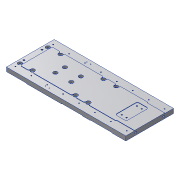
# Autodesk Inventor part: Grundplatte
Saved by Autodesk Inventor 2016 (Build 200138000, 138)
## iProperties
Created: 2015-07-27
Part Number: Grundplatte
Material: Aluminum 6061
Document SubType Name: Modeling
Density: 2.7 g/cm^3
Appearance: Aluminum - Flat
Autodesk Inventor part; units mm, degrees
ref_plane "YZ Plane" through (0, 0, 0) normal (1, 0, 0) x (0, 1, 0)
ref_plane "XZ Plane" through (0, 0, 0) normal (0, 1, 0) x (-1, 0, 0)
ref_plane "XY Plane" through (0, 0, 0) normal (0, 0, 1) x (1, 0, 0)
sketch "Sketch1" plane through (0, 0, 0) normal (0, 0, 1) x (1, 0, 0)
  line L0 (-150, -60) -> (150, -60)
  line L1 (150, -60) -> (150, 60)
  line L2 (150, 60) -> (-150, 60)
  line L3 (-150, 60) -> (-150, -60)
  line L4 (-150, -60) -> (150, 60) construction
  line L5 (150, -60) -> (-150, 60) construction
  point P0 (0, 0)
  dimension "d0" = 300
  dimension "d1" = 120
  constraints: 12 end point, 2 midpoint, 2 parallel, 1 horizontal, 1 perpendicular
  measures "d0" distance of L2.end L1.end
  measures "d1" distance of L1.end L0.end
extrude "Extrusion1" add sketch "Sketch1" along normal blind 12
sketch "Sketch2" plane through (0, 0, 12) normal (0, 0, 1) x (1, 0, 0)
  line L0 (150, -60) -> (-150, -60)
  line L1 (-150, -60) -> (-150, -40)
  line L2 (-150, -40) -> (150, -40)
  line L3 (150, -40) -> (150, -60)
  line L4 (150, 60) -> (-150, 60)
  line L5 (-150, 60) -> (-150, 40)
  line L6 (-150, 40) -> (150, 40)
  line L7 (150, 40) -> (150, 60)
  line L8 (-135, 40) -> (-150, 40)
  line L9 (-150, 40) -> (-150, -40)
  line L10 (-150, -40) -> (-135, -40)
  line L11 (-135, -40) -> (-135, 40)
  line L12 (150, -60) -> (150, 60) projected
  line L13 (-150, -60) -> (150, -60) projected
  line L14 (-150, 60) -> (-150, -60) projected
  line L15 (150, 60) -> (-150, 60) projected
  line L16 (119, 28) -> (91, 28)
  line L17 (91, 28) -> (91, -28)
  line L18 (91, -28) -> (119, -28)
  line L19 (119, -28) -> (119, 28)
  line L20 (150, -40) -> (105, -40)
  line L21 (105, -40) -> (105, -38)
  line L22 (105, -38) -> (150, -38)
  line L23 (150, -38) -> (150, -40)
  line L24 (150, 40) -> (105, 40)
  line L25 (105, 40) -> (105, 38)
  line L26 (105, 38) -> (150, 38)
  line L27 (150, 38) -> (150, 40)
  point P0 (0, 0)
  point P1 (91, 0)
  dimension "d4" = 80
  dimension "d5" = 15
  dimension "d6" = 269
  dimension "d7" = 28
  dimension "d8" = 56
  dimension "d26" = 2
  dimension "d134" = 255
  constraints: 48 end point, 12 parallel, 9 collinear, 6 horizontal, 6 perpendicular, 1 horizontal alignment, 1 midpoint, 1 point on line
  measures "d4" distance between parallel lines of L6 L2
  measures "d5" distance between parallel lines of L9 L11
  measures "d6" distance between parallel lines of L14 L19
  measures "d7" distance of L17.end L18.end
  measures "d8" distance of L18.end L16.start
  measures "d26" distance of L20.end L21.end
  measures "d134" distance between parallel lines of L1 L21
extrude "Extrusion2" cut sketch "Sketch2" against normal blind 1 contours L0 L1 L2 L3 | L2 L21 L22 L12 | L9 L6 L11 L2 | L5 L4 L7 L6 | L26 L25 L6 L12 | L19 L18 L17 L16
fillet "Fillet1" radius 5 4 edges at (119, 28, 11.5) (91, 28, 11.5) (91, -28, 11.5) (119, -28, 11.5)
sketch "Sketch3" plane through (0, 0, 12) normal (0, 0, 1) x (1, 0, 0)
  line L0 (-150, -60) -> (-150, 60) projected
  point P0 (0, 0)
  point P1 (-141, -35)
  point P2 (-109, -35)
  point P3 (-109, 35)
  point P4 (-141, 35)
  point P5 (-1, -35)
  point P6 (31, -35)
  point P7 (31, 35)
  point P8 (-1, 35)
  dimension "d12" = 32
  dimension "d13" = 32
  dimension "d14" = 172
  dimension "d15" = 70
  dimension "d16" = 9
  dimension "d17" = 35
  constraints: 6 horizontal alignment, 4 vertical alignment
  measures "d12" distance of point (-109, -35) point (-141, -35)
  measures "d13" distance of point (31, -35) point (-1, -35)
  measures "d14" distance of point (-141, -35) point (31, -35)
  measures "d15" distance of point (-141, 35) point (-141, -35)
  measures "d16" distance from line of L0 point (-141, -35)
  measures "d17" vertical distance of point (0, 0) point (-141, -35)
hole "Hole1" at (-141, -35, 12) at (-109, -35, 12) at (-109, 35, 12) at (-141, 35, 12) at (-1, -35, 12) at (31, -35, 12) at (31, 35, 12) at (-1, 35, 12) direction (0, 0, -1) diameter 5.5 end through all counterbore diameter 10 counterbore depth 5.7 clearance for "Socket Head Cap Screw ISO 4762" size "M5" standard "ISO"
fillet "Fillet2" radius 3 2 edges at (105, 38, 11.5) (105, -38, 11.5)
sketch "Sketch4" plane through (0, 0, 12) normal (0, 0, 1) x (1, 0, 0)
  circle A0 centre (-109, -35) radius 5 projected
  line L0 (-104, -35) -> (-104, -40)
  line L1 (-104, -40) -> (-114, -40)
  line L2 (-114, -40) -> (-114, -35)
  line L3 (-135, -40) -> (-109, -40) projected
  circle A1 centre (-1, -35) radius 5 projected
  circle A2 centre (31, -35) radius 5 projected
  line L4 (36, -35) -> (36, -40)
  line L5 (36, -40) -> (26, -40)
  line L6 (26, -40) -> (26, -35)
  line L7 (4, -35) -> (4, -40)
  line L8 (4, -40) -> (-6, -40)
  line L9 (-6, -40) -> (-6, -35)
  line L10 (-1, -40) -> (31, -40) projected
  point P0 (0, 0)
  constraints: 18 end point, 6 point on circle, 6 tangent, 5 vertical, 2 collinear, 2 perpendicular, 2 point on line, 1 parallel
extrude "Extrusion3" cut sketch "Sketch4" against normal up to surface (1 mm away) contours L0 L1 A0 | A0 L1 L2 | L7 L8 A1 | A1 L8 L9 | L4 L5 A2 | A2 L5 L6
mirror "Mirror1" about plane through (0, 0, 0) normal (0, 1, 0) of "Extrusion3"
fillet "Fillet3" radius 3 14 edges at (-135, 40, 11.5) (-135, -40, 11.5) (36, 40, 11.5) (26, 40, 11.5) (4, 40, 11.5) (-6, 40, 11.5) (-104, 40, 11.5) (-114, 40, 11.5) (-114, -40, 11.5) (-104, -40, 11.5) (-6, -40, 11.5) (4, -40, 11.5) (26, -40, 11.5) (36, -40, 11.5)
sketch "Sketch5" plane through (0, 0, 11) normal (0, 0, 1) x (1, 0, 0)
  line L0 (-150, -60) -> (-150, 60) projected
  line L1 (-117, 40) -> (-132, 40) projected
  point P0 (0, 0)
  point P1 (-140, 47.5)
  dimension "d31" = 10
  dimension "d32" = 7.5
  measures "d31" distance from line of L0 point (-140, 47.5)
  measures "d32" distance from line of point (-140, 47.5) L1
hole "Hole2" at (-140, 47.5, 11) direction (0, 0, -1) diameter 2.459 end through all thread size "M3x0.5" designation "M3" class "6H" standard "ISO Metric profile"
pattern_linear "Rectangular Pattern1" count 8 spacing 40 along (1, 0, 0) of "Hole2"
mirror "Mirror2" about plane through (0, 0, 0) normal (0, 1, 0) of "Hole2", "Rectangular Pattern1"
sketch "Sketch6" plane through (150, -60, 0) normal (1, 0, 0) x (0, 0, -1)
  line L0 (0, 0) -> (0, 120) projected
  point P0 (0, 60)
  point P1 (-6, 25)
  point P2 (-6, 95)
  dimension "d43" = 70
  dimension "d44" = 35
  dimension "d45" = 6
  constraints: 1 vertical alignment
  measures "d43" distance of point (-6, 95) point (-6, 25)
  measures "d44" vertical distance of point (0, 60) point (-6, 25)
  measures "d45" distance from line of L0 point (-6, 25)
hole "Hole3" at (150, -35, 6) at (150, 35, 6) direction (-1, 0, 0) diameter 4.917 depth 21 tip angle 118 thread size "M6x1" designation "M6" class "6H" standard "ISO Metric profile"
sketch "Sketch7" plane through (0, 0, 11) normal (0, 0, 1) x (1, 0, 0)
  line L0 (-150, -60) -> (-150, 60) projected
  line L1 (-117, 40) -> (-132, 40) projected
  line L2 (-132, -40) -> (-117, -40) projected
  point P0 (0, 0)
  point P1 (-143, 22.5)
  point P2 (-143, -23)
  dimension "d53" = 45.5
  dimension "d54" = 7
  dimension "d55" = 17.5
  dimension "d56" = 17
  constraints: 1 vertical alignment
  measures "d53" distance of point (-143, -23) point (-143, 22.5)
  measures "d54" distance from line of point (-143, 22.5) L0
  measures "d55" distance from line of L1 point (-143, 22.5)
  measures "d56" distance from line of L2 point (-143, -23)
hole "Hole4" at (-143, 22.5, 11) at (-143, -23, 11) direction (0, 0, -1) diameter 4.134 end through all thread size "M5x0.8" designation "M5" class "6H" standard "ISO Metric profile"
sketch "Sketch8" plane through (0, 0, 11) normal (0, 0, 1) x (1, 0, 0)
  line L0 (99, 19) -> (111, 19)
  line L1 (111, 19) -> (111, -19)
  line L2 (111, -19) -> (99, -19)
  line L3 (99, -19) -> (99, 19)
  line L4 (99, 19) -> (111, -19) construction
  line L5 (111, 19) -> (99, -19) construction
  line L6 (91, -23) -> (91, 23) projected
  point P0 (0, 0)
  point P1 (105, 0)
  point P2 (105, 0)
  dimension "d64" = 38
  dimension "d65" = 12
  dimension "d66" = 8
  constraints: 12 end point, 3 midpoint, 2 parallel, 1 horizontal, 1 horizontal alignment, 1 perpendicular
  measures "d64" distance of L2.end L0.start
  measures "d65" distance of L0.start L0.end
  measures "d66" distance between parallel lines of L6 L3
hole "Hole5" at (111, 19, 11) at (99, 19, 11) at (99, -19, 11) at (111, -19, 11) direction (0, 0, -1) diameter 3.242 end through all thread size "M4x0.7" designation "M4" class "6H" standard "ISO Metric profile"
sketch "Sketch9" plane through (0, 0, 12) normal (0, 0, 1) x (1, 0, 0)
  line L0 (-35, 12) -> (-75, 12)
  line L1 (-75, 12) -> (-75, -12)
  line L2 (-75, -12) -> (-35, -12)
  line L3 (-35, -12) -> (-35, 12)
  line L4 (-150, -60) -> (-150, 60) projected
  point P0 (0, 0)
  point P1 (-35, 0)
  dimension "d74" = 24
  dimension "d75" = 40
  dimension "d76" = 75
  constraints: 8 end point, 2 parallel, 1 horizontal, 1 horizontal alignment, 1 midpoint, 1 perpendicular
  measures "d74" distance of L2.end L0.start
  measures "d75" distance of L0.start L0.end
  measures "d76" distance between parallel lines of L4 L1
hole "Hole6" at (-35, 12, 12) at (-35, -12, 12) at (-75, -12, 12) at (-75, 12, 12) direction (0, 0, -1) diameter 5.5 end through all counterbore diameter 10 counterbore depth 5.7 clearance for "Socket Head Cap Screw ISO 4762" size "M5" standard "ISO"
sketch "Sketch10" plane through (0, 0, 0) normal (0, 0, -1) x (-1, 0, 0)
  line L0 (-150, 60) -> (150, 60) projected
  line L1 (150, -60) -> (-150, -60) projected
  line L2 (35, -12) -> (75, -12) construction
  circle A0 centre (35, -12) radius 2.75 projected
  circle A1 centre (75, -12) radius 2.75 projected
  line L3 (50.25, -52) -> (59.75, -52) construction
  point P0 (0, 0)
  point P1 (50.25, 52)
  point P2 (59.75, 52)
  point P3 (55, -52)
  point P4 (55, -12)
  dimension "d84" = 8
  dimension "d85" = 8
  dimension "d86" = 9.5
  constraints: 4 end point, 3 vertical alignment, 2 coincident, 2 horizontal, 2 horizontal alignment, 2 midpoint
  measures "d84" distance from line of L0 point (59.75, 52)
  measures "d85" distance from line of L1 L3.end
  measures "d86" distance of L3.end L3.start
hole "Hole7" at (-50.25, 52, 0) at (-59.75, 52, 0) at (-50.25, -52, 0) at (-59.75, -52, 0) direction (0, 0, 1) diameter 1.567 end through all thread size "M2x0.4" designation "M2" class "6H" standard "ISO Metric profile"
sketch "Sketch11" plane through (-150, 60, 0) normal (0, 1, 0) x (1, 0, 0)
  line L0 (0, 0) -> (0, -11) projected
  line L1 (300, 0) -> (0, 0) projected
  point P0 (150, 0)
  point P1 (5.5, -5)
  point P2 (15, -5)
  dimension "d94" = 5.5
  dimension "d95" = 5
  dimension "d96" = 9.5
  constraints: 1 horizontal alignment
  measures "d94" distance from line of L0 point (5.5, -5)
  measures "d95" distance from line of L1 point (5.5, -5)
  measures "d96" distance of point (15, -5) point (5.5, -5)
hole "Hole8" at (-144.5, 60, 5) at (-135, 60, 5) direction (0, -1, 0) diameter 1.567 depth 10 tip angle 118 thread size "M2x0.4" designation "M2" class "6H" standard "ISO Metric profile"
sketch "Sketch12" plane through (-150, 60, 0) normal (0, 1, 0) x (1, 0, 0)
  line L0 (300, 0) -> (300, -11) projected
  line L1 (300, 0) -> (0, 0) projected
  point P0 (150, 0)
  point P1 (291.5, -5)
  point P2 (282, -5)
  dimension "d104" = 8.5
  dimension "d105" = 9.5
  dimension "d106" = 5
  constraints: 1 horizontal alignment
  measures "d104" distance from line of L0 point (291.5, -5)
  measures "d105" distance of point (282, -5) point (291.5, -5)
  measures "d106" distance from line of L1 point (291.5, -5)
hole "Hole9" at (141.5, 60, 5) at (132, 60, 5) direction (0, -1, 0) diameter 1.567 depth 10 tip angle 118 thread size "M2x0.4" designation "M2" class "6H" standard "ISO Metric profile"
sketch "Sketch13" plane through (0, 0, 12) normal (0, 0, 1) x (1, 0, 0)
  line L0 (105, 60) -> (105, -60)
  line L1 (150, -60) -> (-150, -60) construction
  line L2 (-150, 60) -> (150, 60) construction
  line L3 (-150, -60) -> (-150, 60) construction
  line L4 (105, 60) -> (-150, 60)
  line L5 (-150, 60) -> (-150, -60)
  line L6 (-150, -60) -> (105, -60)
  point P0 (0, 0)
  dimension "d114" = 255
  constraints: 8 end point, 2 perpendicular, 2 point on line, 1 collinear, 1 vertical
  measures "d114" distance between parallel lines of L3 L0
sketch "Sketch14" plane through (0, 0, 0) normal (0, 0, -1) x (-1, 0, 0)
  line L0 (99, 10) -> (150, 10)
  line L1 (150, 10) -> (150, 60)
  line L2 (150, 60) -> (99, 60)
  line L3 (99, 60) -> (99, 10)
  line L4 (-150, 60) -> (150, 60) projected
  line L5 (150, 60) -> (150, -60) projected
  line L6 (-41, 10) -> (11, 10)
  line L7 (11, 10) -> (11, 60)
  line L8 (11, 60) -> (-41, 60)
  line L9 (-41, 60) -> (-41, 10)
  circle A0 centre (-31, 35) radius 2.75 construction
  circle A1 centre (1, 35) radius 2.75 construction
  circle A2 centre (109, 35) radius 2.75 construction
  line L10 (-115, 60) -> (-60, 60)
  line L11 (-60, 60) -> (-60, 50)
  line L12 (-60, 50) -> (-115, 50)
  line L13 (-115, 50) -> (-115, 60)
  point P0 (0, 0)
  dimension "d115" = 50
  dimension "d116" = 51
  dimension "d119" = 52
  dimension "d120" = 10
  dimension "d121" = 10
  dimension "d122" = 10
  dimension "d123" = 10
  dimension "d124" = 55
  dimension "d125" = 265
  constraints: 24 end point, 6 parallel, 3 collinear, 3 horizontal, 3 perpendicular, 2 point on line
  measures "d115" distance of L2.end L0.start
  measures "d116" distance of L0.start L0.end
  measures "d119" distance between parallel lines of L7 L9
  measures "d120" distance from line of A0.centre L9
  measures "d121" distance from line of L7 A1.centre
  measures "d122" distance from line of A2.centre L3
  measures "d123" distance between parallel lines of L4 L12
  measures "d124" distance of L11.end L12.end
  measures "d125" distance between parallel lines of L1 L13
extrude "Extrusion4" cut sketch "Sketch14" against normal blind 1
mirror "Mirror3" about plane through (0, 0, 0) normal (0, 1, 0) of "Extrusion4"
fillet "Fillet4" radius 5 10 edges at (-99, 10, 0.5) (-99, -10, 0.5) (-11, -10, 0.5) (41, -10, 0.5) (-11, 10, 0.5) (41, 10, 0.5) (60, 50, 0.5) (115, 50, 0.5) (115, -50, 0.5) (60, -50, 0.5)
sketch "Sketch15" plane through (0, 0, 0) normal (0, 0, -1) x (-1, 0, 0)
  line L0 (26, -23) -> (84, -23)
  line L1 (84, -23) -> (84, 23)
  line L2 (84, 23) -> (26, 23)
  line L3 (26, 23) -> (26, -23)
  circle A0 centre (35, 12) radius 2.75 construction
  circle A1 centre (75, -12) radius 2.75 construction
  line L4 (75, -12) -> (35, 12) construction
  line L5 (26, 23) -> (84, 23)
  line L6 (84, 23) -> (84, 37)
  line L7 (84, 37) -> (26, 37)
  line L8 (26, 37) -> (26, 23)
  point P0 (0, 0)
  point P1 (55, 23)
  point P2 (55, 0)
  point P3 (26, 0)
  dimension "d127" = 58
  dimension "d128" = 46
  dimension "d130" = 60
  constraints: 18 end point, 4 parallel, 3 midpoint, 2 horizontal, 2 perpendicular, 1 collinear, 1 horizontal alignment, 1 vertical alignment
  measures "d127" distance of L2.end L1.end
  measures "d128" distance of L1.end L0.end
  measures "d130" distance between parallel lines of L0 L7
extrude "Extrusion5" cut sketch "Sketch15" against normal blind 1
fillet "Fillet5" radius 5 4 edges at (-26, -23, 0.5) (-26, 37, 0.5) (-84, 37, 0.5) (-84, -23, 0.5)
equation "\"d17\" = 0.5 * d15"
equation "\"d44\" = 0.5 * d43"
equation "\"d85\" = d84"
equation "\"d114\" = d134"
body "Solid1"
